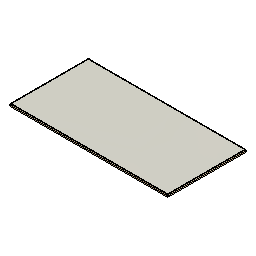
model (Autodesk Fusion 360 design; units mm, degrees)
Autodesk Fusion 360 part; units mm, degrees
sketch "Sketch1" plane through (0, 0, 0) normal (0, 0, 1) x (1, 0, 0)
  line L0 (0, 0) -> (1219.2, 0)
  line L1 (1219.2, 0) -> (1219.2, 609.6)
  line L2 (1219.2, 609.6) -> (0, 609.6)
  line L3 (0, 609.6) -> (0, 0)
  line L4 (10, 10) -> (1209.2, 10)
  line L5 (1209.2, 10) -> (1209.2, 599.6)
  line L6 (1209.2, 599.6) -> (10, 599.6)
  line L7 (10, 599.6) -> (10, 10)
  line L8 (10, 599.6) -> (0, 609.6)
  line L9 (1209.2, 599.6) -> (1219.2, 609.6)
  line L10 (1209.2, 10) -> (1219.2, 0)
  line L11 (0, 0) -> (10, 10)
  arc A0 (0, 10) -> (10, 0) centre (10, 10) ccw
  arc A1 (10, 609.6) -> (0, 599.6) centre (10, 599.6) ccw
  arc A2 (1219.2, 599.6) -> (1209.2, 609.6) centre (1209.2, 599.6) ccw
  arc A3 (1209.2, 0) -> (1219.2, 10) centre (1209.2, 10) ccw
  dimension "d1" = 1219.2
  dimension "d2" = 609.6
  dimension "d3" = -10
  dimension "d10" = 10
  constraint horizontal L0
  constraint vertical L1
  constraint horizontal L2
  constraint vertical L3
  constraint coincident L0.start L3.end
  constraint tangent L0 A0
  constraint coincident L0 A0.end
  constraint coincident L3 A0.start
  constraint tangent L3 A0
  constraint coincident L4.start L7.end
  constraint coincident L2 A1.start
  constraint coincident L3 A1.end
  constraint coincident L6.end L7.start
  constraint coincident L1 A2.start
  constraint coincident L2 A2.end
  constraint coincident L5.end L6.start
  constraint coincident L0 A3.start
  constraint coincident L1 A3.end
  constraint coincident L4.end L5.start
  constraint tangent L0 A3
  constraint tangent L2 A2
  constraint tangent L3 A1
  measures "d1" distance of L1.end L2.end
  measures "d2" distance of L0.end L1.end
  measures "d10" radius of A0
extrude "Extrude1" add sketch "Sketch1" along normal blind 19.05 contours L4 L5 L6 L7 makes body 1
extrude "Extrude2" add sketch "Sketch1" along normal up to surface (19.05 mm away) separate body contours L3 L7 L8 L11 A0 A1 | L1 L5 L9 L10 A2 A3 makes body 2 at (0, 403.0667, 12.7) makes body 3 at (1209.2, 206.5333, 12.7)
extrude "Extrude3" add sketch "Sketch1" along normal up to surface (19.05 mm away) separate body contours L0 L4 L10 L11 A0 A3 | L2 L6 L8 L9 A1 A2 makes body 4 at (409.7333, 10, 6.35) makes body 5 at (809.4667, 609.6, 6.35)
chamfer "Chamfer1" distance 5 angle 45 12 edges at (609.6, 0, 0) (1213.0268, 0.7612, 0) (6.1732, 0.7612, 0) (609.6, 609.6, 0) (6.1732, 608.8388, 0) (1213.0268, 608.8388, 0) (1219.2, 304.8, 0) (1218.4388, 603.4268, 0) (1218.4388, 6.1732, 0) (0, 304.8, 0) (0.7612, 6.1732, 0) (0.7612, 603.4268, 0) on bodies 2 3 4 5
fillet "Fillet1" radius 4.7625 12 edges at (0.7612, 6.1732, 19.05) (0, 304.8, 19.05) (0.7612, 603.4268, 19.05) (1218.4388, 603.4268, 19.05) (1219.2, 304.8, 19.05) (1218.4388, 6.1732, 19.05) (1213.0268, 0.7612, 19.05) (609.6, 0, 19.05) (6.1732, 0.7612, 19.05) (6.1732, 608.8388, 19.05) (609.6, 609.6, 19.05) (1213.0268, 608.8388, 19.05) on bodies 2 3 4 5
equation "d1 = 4'-0\""
equation "d2 = 2'-0\""
equation "d4 = 3/4\""
equation "d13 = 3/16\""
